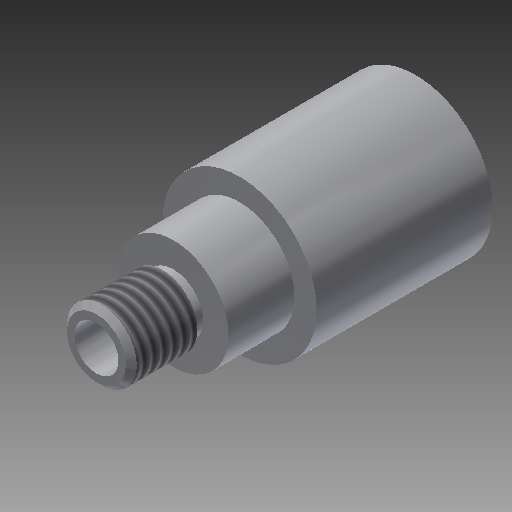
# Autodesk Inventor part: Gewindeadapter
Saved by Autodesk Inventor 2018 (Build 220112000, 112)
## iProperties
Created: 2013-03-06
Part Number: Gewindeadapter
Material: Aluminum-6061
Document SubType Name: Modeling
Designer: Neef
Mass: 5.70524 g
Surface Area: 18.8365 cm^2
Volume: 2.11305 cm^3
Density: 2.7 g/cm^3
Appearance: Aluminum - Flat
Author: Neef
Autodesk Inventor part; units mm, degrees
ref_plane "YZ Plane" through (0, 0, 0) normal (1, 0, 0) x (0, 1, 0)
ref_plane "XZ Plane" through (0, 0, 0) normal (0, 1, 0) x (-1, 0, 0)
ref_plane "XY Plane" through (0, 0, 0) normal (0, 0, 1) x (1, 0, 0)
sketch "Skizze1" plane through (0, 0, 0) normal (0, 0, 1) x (1, 0, 0)
  line L0 (0, 34.8) -> (0, -5.8) projected
  line L1 (-1.4, 0) -> (8.4, 0) projected
  line L2 (2, 0) -> (2, 16)
  line L3 (2, 16) -> (4.5, 16)
  line L4 (4.5, 16) -> (4.5, 29)
  line L5 (4.5, 29) -> (7, 29)
  line L6 (7, 29) -> (7, 13)
  line L7 (3.175, 6) -> (3.175, 0)
  line L8 (2, 0) -> (3.175, 0)
  line L9 (5, 7) -> (2.7, 7)
  line L10 (2.7, 7) -> (2.7, 6)
  line L11 (2.7, 6) -> (3.175, 6)
  line L12 (7, 13) -> (5, 13)
  line L13 (5, 13) -> (5, 7)
  point P0 (0, 0)
  dimension "d1" = 1
  dimension "d2" = 2.7
  dimension "d3" = 3.175
  dimension "d4" = 2
  dimension "d5" = 4.5
  dimension "d6" = 13
  dimension "d7" = 7
  dimension "d8" = 5
  dimension "d9" = 6
  dimension "d10" = 3
  dimension "d11" = 7
  constraints: 24 end point, 8 perpendicular, 3 parallel, 2 point on line, 1 collinear
  measures "d1" distance of L9.end L10.end
  measures "d2" distance between parallel lines of L0 L10
  measures "d3" distance between parallel lines of L0 L7
  measures "d4" distance between parallel lines of L0 L2
  measures "d5" distance between parallel lines of L0 L4
  measures "d6" distance of L3.end L4.end
  measures "d7" distance between parallel lines of L0 L6
  measures "d8" distance between parallel lines of L0 L13
  measures "d9" distance of L12.end L9.start
  measures "d10" distance between parallel lines of L12 L3
  measures "d11" distance between parallel lines of L1 L9
revolve "Umdrehung1" add sketch "Skizze1" angle 360 about axis through (0, 0, 0) along (0, -1, 0)
chamfer "Fase1" distance 0.5 angle 45 2 edges at (-3.175, 0, 0) (-4.5, 29, 0)
thread "Gewinde1" size "G9.728x0.907" designation "G 1/8" standard "ISO Pipe Threads" full length
thread "Gewinde2" size "1/4-28 UNF" class "2A" standard "ANSI Unified Screw Threads" full length
